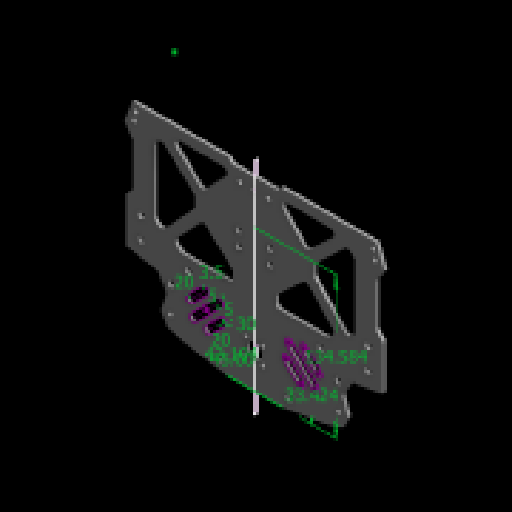
# Autodesk Inventor part: HeadMount
Saved by Autodesk Inventor 2025.2 (Build 292293000, 293)
## iProperties
Created: 2024-12-17
Part Number: HeadMount
Material: Generic
Document SubType Name: Sheet Metal
Designer: valer
Density: 1 g/cm^3
Sheet Metal Rule: Default
Appearance: Default
Author: valer
Autodesk Inventor part; units mm, degrees
ref_plane "YZ Plane" through (0, 0, 0) normal (1, 0, 0) x (0, 1, 0)
ref_plane "XZ Plane" through (0, 0, 0) normal (0, 1, 0) x (-1, 0, 0)
ref_plane "XY Plane" through (0, 0, 0) normal (0, 0, 1) x (1, 0, 0)
sketch "Sketch1" plane through (0, 0, 0) normal (0, 0, 1) x (1, 0, 0)
  circle A0 centre (-31.8464, -169.787) radius 2.7 construction
  circle A1 centre (-31.8464, -149.787) radius 2.7 construction
  arc A2 (-25.8464, -149.787) -> (-31.8464, -143.787) centre (-31.8464, -149.787) ccw construction
  line L0 (-31.8464, -143.787) -> (-53.675, -143.787) construction
  line L1 (-56.8232, -161.2642) -> (-53.675, -143.787) construction
  line L2 (-55.3879, -175.787) -> (-56.8232, -161.2642) construction
  line L3 (-55.3879, -175.787) -> (-31.8464, -175.787) construction
  arc A3 (-31.8464, -175.787) -> (-25.8464, -169.787) centre (-31.8464, -169.787) ccw construction
  line L4 (-25.8464, -169.787) -> (-25.8464, -149.787) construction
  circle A4 centre (183.4534, -169.787) radius 2.7 construction
  circle A5 centre (183.4534, -149.787) radius 2.7 construction
  arc A6 (183.4534, -143.787) -> (177.4534, -149.787) centre (183.4534, -149.787) ccw construction
  line L5 (177.4534, -169.787) -> (177.4534, -149.787) construction
  arc A7 (177.4534, -169.787) -> (183.4534, -175.787) centre (183.4534, -169.787) ccw construction
  line L6 (206.995, -175.787) -> (183.4534, -175.787) construction
  line L7 (206.995, -175.787) -> (208.4302, -161.2642) construction
  line L8 (208.4302, -161.2642) -> (205.282, -143.787) construction
  line L9 (183.4534, -143.787) -> (205.282, -143.787) construction
  line L10 (75.8035, -414.1995) -> (75.8035, 156.7514) construction
  line L11 (-46.34, -181.787) -> (-13.5242, -244.787)
  line L12 (-68.027, -161.7986) -> (-24.4397, -245.4777) construction
  line L13 (22.7981, -247.6758) -> (7.7102, -247.6758) construction
  circle A8 centre (22.7981, -241.6758) radius 2.7 construction
  circle A9 centre (22.7981, -223.6758) radius 2.7 construction
  circle A10 centre (22.7981, -223.6758) radius 3
  circle A11 centre (22.7981, -241.6758) radius 3
  circle A12 centre (-31.8464, -169.787) radius 3
  circle A13 centre (-31.8464, -149.787) radius 3
  line L14 (50.5095, -95.6646) -> (64.5095, -80.8626) construction
  line L15 (58.6334, -80.1159) -> (70.8035, -80.1159) construction
  circle A14 centre (37.042, -105.0395) radius 2.7 construction
  circle A15 centre (37.042, -117.0395) radius 2.7 construction
  circle A16 centre (114.5651, -105.0395) radius 2.7 construction
  circle A17 centre (114.5651, -117.0395) radius 2.7 construction
  circle A18 centre (128.8089, -223.6758) radius 2.7 construction
  circle A19 centre (128.8089, -241.6758) radius 2.7 construction
  line L16 (49.1565, -240.3427) -> (18.4758, -250.5451)
  line L17 (18.4758, -250.5451) -> (-13.5242, -244.787)
  line L18 (-39.6272, -91.7884) -> (-39.6272, -131.787)
  line L19 (-39.6272, -131.787) -> (-46.34, -139.787)
  line L20 (-46.34, -139.787) -> (-46.34, -181.787)
  line L21 (197.9471, -181.787) -> (165.1312, -244.787)
  circle A20 centre (128.8089, -223.6758) radius 3
  circle A21 centre (128.8089, -241.6758) radius 3
  circle A22 centre (183.4534, -169.787) radius 3
  circle A23 centre (183.4534, -149.787) radius 3
  line L22 (102.4505, -240.3427) -> (133.1312, -250.5451)
  line L23 (133.1312, -250.5451) -> (165.1312, -244.787)
  line L24 (191.2343, -91.7884) -> (191.2343, -131.787)
  line L25 (191.2343, -131.787) -> (197.9471, -139.787)
  line L26 (197.9471, -139.787) -> (197.9471, -181.787)
  circle A24 centre (-36.9593, -67.1208) radius 1.75 construction
  circle A25 centre (-38.635, -75.4158) radius 1.75 construction
  line L27 (-49.4079, -79.3835) -> (-42.2489, -59.9463) construction
  line L28 (-38.8427, -81.4928) -> (-49.4079, -79.3835) construction
  line L29 (-34.1095, -78.2645) -> (-38.8427, -81.4928) construction
  line L30 (-31.6784, -66.23) -> (-34.1095, -78.2645) construction
  line L31 (-34.7908, -61.4353) -> (-31.6784, -66.23) construction
  line L32 (-42.2489, -59.9463) -> (-34.7908, -61.4353) construction
  circle A26 centre (188.5664, -67.1208) radius 1.75 construction
  circle A27 centre (190.2421, -75.4158) radius 1.75 construction
  line L33 (193.8559, -59.9463) -> (201.0149, -79.3835) construction
  line L34 (186.3979, -61.4353) -> (193.8559, -59.9463) construction
  line L35 (183.2854, -66.23) -> (186.3979, -61.4353) construction
  line L36 (185.7165, -78.2645) -> (183.2854, -66.23) construction
  line L37 (190.4497, -81.4928) -> (185.7165, -78.2645) construction
  line L38 (201.0149, -79.3835) -> (190.4497, -81.4928) construction
  line L39 (-39.6272, -91.7884) -> (-47.4225, -79.7798)
  line L40 (-47.4225, -79.7798) -> (-40.2635, -60.3427)
  line L41 (-40.2635, -60.3427) -> (75.8035, -60.3427)
  line L42 (191.2343, -91.7884) -> (199.0296, -79.7798)
  line L43 (199.0296, -79.7798) -> (191.8706, -60.3427)
  line L44 (191.8706, -60.3427) -> (75.8035, -60.3427)
  line L45 (49.1565, -240.3427) -> (102.4505, -240.3427)
  circle A28 centre (-38.635, -75.4158) radius 2
  circle A29 centre (-36.9593, -67.1208) radius 2
  circle A30 centre (188.5664, -67.1208) radius 2
  circle A31 centre (190.2421, -75.4158) radius 2
  line L46 (-46.34, -181.787) -> (-15.2365, -187.3838)
  line L47 (-15.2365, -187.3838) -> (8.958, -233.8324)
  line L48 (8.958, -233.8324) -> (8.958, -248.8324)
  line L49 (197.9471, -181.787) -> (166.8435, -187.3838)
  line L50 (166.8435, -187.3838) -> (142.6491, -233.8324)
  line L51 (142.6491, -233.8324) -> (142.6491, -248.8324)
  line L52 (8.958, -233.8324) -> (49.1565, -240.3427)
  line L53 (102.4505, -240.3427) -> (142.6491, -233.8324)
  line L54 (142.6491, -233.8324) -> (158.8354, -228.7333)
  line L55 (158.8354, -228.7333) -> (164.3791, -218.0906)
  line L56 (164.3791, -218.0906) -> (159.28, -201.9042)
  line L57 (161.6073, -223.412) -> (150.9645, -217.8683) construction
  line L58 (8.958, -233.8324) -> (-7.2284, -228.7333)
  line L59 (-7.2284, -228.7333) -> (-12.7721, -218.0906)
  line L60 (-12.7721, -218.0906) -> (-7.673, -201.9042)
  point P0 (0, 0)
  point P1 (29.3253, -99.0395)
  point P2 (-39.6272, -132.4563)
  point P3 (-39.6272, -132.4563)
  dimension "d6" = 6
  dimension "d7" = 6
  dimension "d8" = 6
  dimension "d9" = 6
  dimension "d32" = 10
  dimension "d51" = 140
  dimension "d58" = 8
  dimension "d69" = 63
  dimension "d73" = 42
  dimension "d82" = 32
  dimension "d209" = 2
  dimension "d210" = 4
  dimension "d211" = 4
  dimension "d212" = 4
  dimension "d213" = 4
  dimension "d238" = 6
  dimension "d239" = 71.606
  dimension "d240" = 151.406
  dimension "d241" = 180
  dimension "d262" = 25
  dimension "d263" = 15
  dimension "d264" = 45
  dimension "d265" = 12
  dimension "d266" = 12
  measures "d6" diameter of A10
  measures "d7" diameter of A11
  measures "d8" diameter of A12
  measures "d9" diameter of A13
  measures "d32" distance between parallel lines of L11 L12
  measures "d51" angle of L20 L19
  measures "d58" vertical distance of L18.end L19.end
  measures "d69" vertical distance of L11.start L11.end
  measures "d73" distance of L19.end L11.start
  measures "d82" horizontal distance of L16.end L11.end
  measures "d209" distance between parallel lines of L27 L40
  measures "d210" diameter of A28
  measures "d211" diameter of A29
  measures "d212" diameter of A30
  measures "d213" diameter of A31
  measures "d238" distance from line of L3 L11.start
  measures "d239" angle of L16 L10
  measures "d240" angle of L16 L17
  measures "d241" distance between parallel lines of L45 L41
  measures "d262" distance between parallel lines of L11 L47
  measures "d263" distance of L47.end L48.end
  measures "d264" angle of L50 L54
  measures "d265" distance of L57.start L57.end
  measures "d266" distance of L54.end L55.end
extrude "Plate1" add sketch "Sketch1" along normal blind 3 contours L20 L19 L18 L39 L40 L41 L44 L43 L42 L24 L25 L26 L49 L50 L53 L45 L52 L47 L46 | L47 L58 L59 L60 | L50 L56 L55 L54 | A10 | A20
sketch "Sketch10" plane through (0, 0, 3) normal (0, 0, 1) x (1, 0, 0)
  arc A0 (76.8035, -214.1927) -> (74.8035, -214.1927) centre (75.8035, -207.2645) ccw construction
  circle A1 centre (75.8035, -207.2645) radius 7
  line L0 (45.7546, -229.3135) -> (45.0245, -232.0574) construction
  arc A2 (45.7546, -229.3135) -> (45.0245, -232.0574) centre (42.9736, -230.0426) ccw construction
  arc A3 (106.1334, -231.4623) -> (106.1334, -228.6229) centre (108.6334, -230.0426) ccw construction
  circle A4 centre (42.9736, -230.0426) radius 3.1
  circle A5 centre (108.6334, -230.0426) radius 3.1
  arc A6 (-1.2619, -190.9216) -> (-1.2619, -193.761) centre (-3.7619, -192.3413) ccw construction
  arc A7 (15.5855, -171.9674) -> (15.5855, -174.8068) centre (13.0855, -173.3871) ccw construction
  arc A8 (136.0216, -174.8068) -> (136.0216, -171.9674) centre (138.5216, -173.3871) ccw construction
  arc A9 (152.8689, -193.761) -> (152.8689, -190.9216) centre (155.3689, -192.3413) ccw construction
  arc A10 (-1.2619, -190.9216) -> (-1.2619, -193.761) centre (-3.7619, -192.3413) ccw projected
  circle A11 centre (-3.7619, -192.3413) radius 3.1
  arc A12 (15.5855, -171.9674) -> (15.5855, -174.8068) centre (13.0855, -173.3871) ccw projected
  circle A13 centre (13.0855, -173.3871) radius 3.1
  arc A14 (136.0216, -174.8068) -> (136.0216, -171.9674) centre (138.5216, -173.3871) ccw projected
  circle A15 centre (138.5216, -173.3871) radius 3.1
  circle A16 centre (155.3689, -192.3413) radius 3.1
  arc A17 (69.2244, -198.4257) -> (66.5765, -198.1614) centre (67.8035, -199.2645) ccw construction
  arc A18 (85.7112, -198.6639) -> (85.5795, -200.1843) centre (83.8035, -199.2645) ccw construction
  arc A19 (65.8958, -215.8651) -> (66.0276, -214.3447) centre (67.8035, -215.2645) ccw construction
  arc A20 (84.4041, -217.1722) -> (82.8838, -217.0405) centre (83.8035, -215.2645) ccw construction
  circle A21 centre (67.8035, -199.2645) radius 2.1
  circle A22 centre (83.8035, -199.2645) radius 2.1
  circle A23 centre (83.8035, -215.2645) radius 2.1
  circle A24 centre (67.8035, -215.2645) radius 2.1
  point P0 (0, 0)
  dimension "d150" = 6.2
  dimension "d153" = 4.2
  constraints: 11 coincident, 10 centre point, 8 equal radius, 3 other
  measures "d150" diameter of A4
  measures "d153" diameter of A21
extrude "Extrusion5" cut sketch "Sketch10" against normal through all
sketch "Sketch11" plane through (0, 0, 3) normal (0, 0, 1) x (1, 0, 0)
  line L0 (42.8154, -184.2567) -> (17.679, -209.3932) construction
  line L1 (40.3405, -181.7819) -> (15.2041, -206.9183)
  line L2 (20.1538, -211.868) -> (45.2903, -186.7316)
  arc A0 (45.2903, -186.7316) -> (40.3405, -181.7819) centre (42.8154, -184.2567) ccw
  arc A1 (15.2041, -206.9183) -> (20.1538, -211.868) centre (17.679, -209.3932) ccw
  line L3 (45.8035, -198.2392) -> (31.6614, -212.3813) construction
  line L4 (43.3286, -195.7643) -> (29.1865, -209.9064)
  line L5 (34.1363, -214.8562) -> (48.2784, -200.714)
  arc A2 (48.2784, -200.714) -> (43.3286, -195.7643) centre (45.8035, -198.2392) ccw
  arc A3 (29.1865, -209.9064) -> (34.1363, -214.8562) centre (31.6614, -212.3813) ccw
  line L6 (28.833, -181.2686) -> (14.6908, -195.4107) construction
  line L7 (31.3078, -183.7435) -> (17.1657, -197.8856)
  line L8 (12.2159, -192.9359) -> (26.3581, -178.7937)
  arc A4 (31.3078, -183.7435) -> (26.3581, -178.7937) centre (28.833, -181.2686) ccw
  arc A5 (12.2159, -192.9359) -> (17.1657, -197.8856) centre (14.6908, -195.4107) ccw
  line L9 (75.8035, -105.7591) -> (75.8035, -240.3427) construction
  line L10 (21.7619, -188.3397) -> (38.7325, -205.3102) construction
  line L11 (111.2665, -181.7819) -> (136.403, -206.9183)
  line L12 (131.4532, -211.868) -> (106.3168, -186.7316)
  arc A6 (111.2665, -181.7819) -> (106.3168, -186.7316) centre (108.7917, -184.2567) ccw
  arc A7 (131.4532, -211.868) -> (136.403, -206.9183) centre (133.9281, -209.3932) ccw
  line L13 (108.2784, -195.7643) -> (122.4205, -209.9064)
  line L14 (117.4708, -214.8562) -> (103.3286, -200.714)
  arc A8 (108.2784, -195.7643) -> (103.3286, -200.714) centre (105.8035, -198.2392) ccw
  arc A9 (117.4708, -214.8562) -> (122.4205, -209.9064) centre (119.9457, -212.3813) ccw
  line L15 (120.2992, -183.7435) -> (134.4413, -197.8856)
  line L16 (139.3911, -192.9359) -> (125.249, -178.7937)
  arc A10 (125.249, -178.7937) -> (120.2992, -183.7435) centre (122.7741, -181.2686) ccw
  arc A11 (134.4413, -197.8856) -> (139.3911, -192.9359) centre (136.9162, -195.4107) ccw
  line L17 (102.4505, -240.3427) -> (49.1565, -240.3427) projected
  point P0 (0, 0)
  point P1 (30.2472, -196.8249)
  dimension "d154" = 3.5
  dimension "d155" = 5
  dimension "d156" = 5
  dimension "d163" = 30
  dimension "d165" = 20
  dimension "d214" = 45
  dimension "d215" = 42.1035
  dimension "d217" = 33.4244
  dimension "d218" = 134.5835
  dimension "d242" = 20
  constraints: 40 end point, 24 point on circle, 18 symmetric about line, 12 centre point, 12 tangent, 5 midpoint, 5 parallel, 2 equal radius, 2 perpendicular, 6 other
  measures "d154" radius of A4
  measures "d155" distance between parallel lines of L1 L7
  measures "d156" distance between parallel lines of L4 L2
  measures "d163" distance from line of L9 L3.start
  measures "d165" distance of L6.start L6.end
  measures "d214" angle of L17 L3
  measures "d215" distance from line of L17 L3.start
  measures "d217" distance from line of L11.end L17
  measures "d218" distance from line of L9.start L17
  measures "d242" distance of L3.start L3.end
extrude "Extrusion6" cut sketch "Sketch11" against normal through all
sketch "Sketch13" plane through (0, 0, 3) normal (0, 0, 1) x (1, 0, 0)
  circle A0 centre (62.3035, -56.7429) radius 2 construction
  circle A1 centre (89.3035, -56.7429) radius 2 construction
  line L0 (98.1778, -70.2429) -> (53.4293, -70.2429) construction
  line L1 (75.8035, -70.2429) -> (75.8035, -80.2429) construction
  line L2 (53.4293, -70.2429) -> (53.4293, -80.2429) construction
  line L3 (53.4293, -75.2429) -> (75.8035, -75.2429) construction
  line L4 (62.3035, -56.7429) -> (62.3035, -75.2429) construction
  circle A2 centre (62.3035, -75.2429) radius 2
  circle A3 centre (75.8035, -75.2429) radius 2
  circle A4 centre (89.3035, -75.2429) radius 2
  point P0 (0, 0)
  dimension "d174" = 4
  dimension "d175" = 4
  constraints: 10 end point, 3 centre point, 3 midpoint, 2 coincident, 1 perpendicular, 1 point on line, 1 symmetric about line, 1 vertical, 1 other
  measures "d174" diameter of A2
  measures "d175" diameter of A3
extrude "Cut1" cut sketch "Sketch13" against normal blind 3
fillet "Fillet1" radius 2 20 edges at (-39.6272, -91.7884, 1.5) (-39.6272, -131.787, 1.5) (-46.34, -139.787, 1.5) (-46.34, -181.787, 1.5) (49.1565, -240.3427, 1.5) (102.4505, -240.3427, 1.5) (197.9471, -181.787, 1.5) (197.9471, -139.787, 1.5) (191.2343, -131.787, 1.5) (191.2343, -91.7884, 1.5) (-15.2365, -187.3838, 1.5) (8.958, -233.8324, 1.5) (166.8435, -187.3838, 1.5) (142.6491, -233.8324, 1.5) (-7.673, -201.9042, 1.5) (-12.7721, -218.0906, 1.5) (-7.2284, -228.7333, 1.5) (159.28, -201.9042, 1.5) (164.3791, -218.0906, 1.5) (158.8354, -228.7333, 1.5)
sketch "Sketch17" plane through (0, 0, 3) normal (0, 0, 1) x (1, 0, 0)
  line L0 (44.5586, -95.6074) -> (52.8519, -81.2429)
  arc A0 (54.584, -80.2429) -> (52.8519, -81.2429) centre (54.584, -82.2429) ccw
  line L1 (54.584, -80.2429) -> (97.023, -80.2429)
  arc A1 (98.7551, -81.2429) -> (97.023, -80.2429) centre (97.023, -82.2429) ccw
  line L2 (98.7551, -81.2429) -> (107.0485, -95.6074)
  arc A2 (107.269, -97.0403) -> (107.0485, -95.6074) centre (105.3164, -96.6074) ccw
  line L3 (106.3291, -101.28) -> (107.269, -97.0403)
  arc A3 (105.5236, -102.4855) -> (106.3291, -101.28) centre (104.3765, -100.8471) ccw
  line L4 (105.5236, -102.4855) -> (98.5318, -107.3812)
  arc A4 (97.3847, -107.7429) -> (98.5318, -107.3812) centre (97.3847, -105.7429) ccw
  line L5 (97.3847, -107.7429) -> (54.2224, -107.7429)
  arc A5 (53.0752, -107.3812) -> (54.2224, -107.7429) centre (54.2224, -105.7429) ccw
  line L6 (53.0752, -107.3812) -> (46.0834, -102.4855)
  arc A6 (45.278, -101.28) -> (46.0834, -102.4855) centre (47.2306, -100.8471) ccw
  line L7 (44.338, -97.0403) -> (45.278, -101.28)
  arc A7 (44.5586, -95.6074) -> (44.338, -97.0403) centre (46.2906, -96.6074) ccw
  point P0 (0, 0)
sheet face with bend "Face6" sketch "Sketch17" thickness 3 toward (0, 0, -1) bend radius 3 relief straight relief width 3 relief depth 1.5
bend "Bend5"
sketch "Sketch18" plane through (0, 0, 3) normal (0, 0, 1) x (1, 0, 0)
  line L0 (4.6693, -117.8173) -> (9.4448, -115.0601)
  arc A0 (10.4448, -114.7922) -> (9.4448, -115.0601) centre (10.4448, -116.7922) ccw
  line L1 (10.4448, -114.7922) -> (17.373, -114.7922)
  arc A1 (18.373, -115.0601) -> (17.373, -114.7922) centre (17.373, -116.7922) ccw
  arc A2 (4.6693, -117.8173) -> (3.7838, -118.8824) centre (5.6693, -119.5493) ccw
  line L2 (3.7838, -118.8824) -> (2.248, -123.2238)
  arc A3 (2.248, -123.2238) -> (2.2668, -124.6088) centre (4.1335, -123.8908) ccw
  line L3 (16.2921, -161.0744) -> (2.2668, -124.6088)
  line L4 (18.373, -115.0601) -> (45.611, -130.786)
  arc A4 (46.611, -132.5181) -> (45.611, -130.786) centre (44.611, -132.5181) ccw
  line L5 (46.611, -132.5181) -> (46.611, -148.4861)
  arc A5 (46.611, -148.4861) -> (47.2565, -149.9575) centre (48.611, -148.4861) ccw
  line L6 (47.2565, -149.9575) -> (59.7731, -161.4802)
  arc A6 (60.4142, -163.082) -> (59.7731, -161.4802) centre (58.4185, -162.9516) ccw
  line L7 (60.4142, -163.082) -> (59.8495, -171.7285)
  arc A7 (59.3252, -172.9527) -> (59.8495, -171.7285) centre (57.8538, -171.5981) ccw
  line L8 (59.3252, -172.9527) -> (57.0902, -175.3806)
  arc A8 (55.7014, -176.0243) -> (57.0902, -175.3806) centre (55.6187, -174.026) ccw
  line L9 (51.7048, -176.1895) -> (55.7014, -176.0243)
  arc A9 (50.2676, -175.6627) -> (51.7048, -176.1895) centre (51.6222, -174.1912) ccw
  line L10 (50.2676, -175.6627) -> (39.6798, -165.9157)
  arc A10 (39.6798, -165.9157) -> (38.3252, -165.3871) centre (38.3252, -167.3871) ccw
  line L11 (38.3252, -165.3871) -> (22.5715, -165.3871)
  arc A11 (21.4392, -165.0357) -> (22.5715, -165.3871) centre (22.5715, -163.3871) ccw
  line L12 (17.0265, -162.0051) -> (21.4392, -165.0357)
  arc A12 (16.2921, -161.0744) -> (17.0265, -162.0051) centre (18.1588, -160.3565) ccw
  arc A13 (91.834, -161.4802) -> (91.1928, -163.082) centre (93.1886, -162.9516) ccw
  line L13 (91.834, -161.4802) -> (104.3506, -149.9575)
  line L14 (91.7575, -171.7285) -> (91.1928, -163.082)
  arc A14 (91.7575, -171.7285) -> (92.2818, -172.9527) centre (93.7532, -171.5981) ccw
  line L15 (94.5169, -175.3806) -> (92.2818, -172.9527)
  arc A15 (94.5169, -175.3806) -> (95.9057, -176.0243) centre (95.9883, -174.026) ccw
  line L16 (95.9057, -176.0243) -> (99.9023, -176.1895)
  arc A16 (99.9023, -176.1895) -> (101.3395, -175.6627) centre (99.9849, -174.1912) ccw
  line L17 (111.9273, -165.9157) -> (101.3395, -175.6627)
  arc A17 (113.2818, -165.3871) -> (111.9273, -165.9157) centre (113.2818, -167.3871) ccw
  line L18 (129.0355, -165.3871) -> (113.2818, -165.3871)
  arc A18 (129.0355, -165.3871) -> (130.1678, -165.0357) centre (129.0355, -163.3871) ccw
  line L19 (130.1678, -165.0357) -> (134.5805, -162.0051)
  arc A19 (134.5805, -162.0051) -> (135.3149, -161.0744) centre (133.4482, -160.3565) ccw
  line L20 (149.3402, -124.6088) -> (135.3149, -161.0744)
  arc A20 (149.3402, -124.6088) -> (149.359, -123.2238) centre (147.4735, -123.8908) ccw
  line L21 (149.359, -123.2238) -> (147.8233, -118.8824)
  arc A21 (147.8233, -118.8824) -> (146.9378, -117.8173) centre (145.9378, -119.5493) ccw
  line L22 (142.1622, -115.0601) -> (146.9378, -117.8173)
  arc A22 (142.1622, -115.0601) -> (141.1622, -114.7922) centre (141.1622, -116.7922) ccw
  line L23 (134.234, -114.7922) -> (141.1622, -114.7922)
  arc A23 (134.234, -114.7922) -> (133.234, -115.0601) centre (134.234, -116.7922) ccw
  line L24 (105.996, -130.786) -> (133.234, -115.0601)
  arc A24 (105.996, -130.786) -> (104.996, -132.5181) centre (106.996, -132.5181) ccw
  line L25 (104.996, -148.4861) -> (104.996, -132.5181)
  arc A25 (104.3506, -149.9575) -> (104.996, -148.4861) centre (102.996, -148.4861) ccw
  point P0 (0, 0)
sheet face with bend "Face7" sketch "Sketch18" thickness 3 toward (0, 0, -1) bend radius 3 relief straight relief width 3 relief depth 1.5
bend "Bend6"
sketch "Sketch19" plane through (0, 0, 3) normal (0, 0, 1) x (1, 0, 0)
  line L0 (191.8706, -60.3427) -> (-40.2635, -60.3427) projected
  line L1 (50.9033, -60.3427) -> (54.8035, -64.2429)
  line L2 (54.8035, -64.2429) -> (96.8035, -64.2429)
  line L3 (96.8035, -64.2429) -> (100.7037, -60.3427)
  line L4 (75.8035, -64.2429) -> (75.8035, -60.3427)
  line L5 (-40.2635, -60.3427) -> (191.8706, -60.3427) projected
  line L6 (96.8035, -64.2429) -> (54.8035, -64.2429) projected
  point P0 (0, 0)
  constraints: 8 end point, 3 perpendicular, 2 midpoint, 2 point on line, 1 collinear, 1 parallel
extrude "Cut3" cut sketch "Sketch19" against normal blind 3
sketch "Sketch20" plane through (0, 0, 3) normal (0, 0, 1) x (1, 0, 0)
  line L0 (-5.9873, -70.3427) -> (54.8035, -70.3427)
  line L1 (54.8035, -70.3427) -> (26.5284, -100.664)
  line L2 (-5.9873, -70.3427) -> (26.5284, -100.664)
  line L3 (19.7084, -107.9776) -> (19.7084, -117.9776)
  line L4 (19.7084, -117.9776) -> (-12.3137, -152.3171)
  line L5 (54.8035, -64.2429) -> (50.9033, -60.3427) projected
  line L6 (-40.2635, -60.3427) -> (50.9033, -60.3427) projected
  line L7 (-39.6272, -131.059) -> (-39.6272, -92.3806) projected
  line L8 (-46.34, -180.1147) -> (-46.34, -140.5149) projected
  line L9 (-45.8721, -139.2293) -> (-40.0951, -132.3446) projected
  line L10 (-39.9497, -91.2916) -> (-47.4225, -79.7798) projected
  line L11 (-47.4225, -79.7798) -> (-40.2635, -60.3427) projected
  line L12 (-0.9715, -154.8168) -> (27.022, -124.7976)
  line L13 (55.8035, -161.6368) -> (6.3421, -161.6368)
  line L14 (6.3421, -161.6368) -> (-0.9715, -154.8168)
  line L15 (27.022, -124.7976) -> (55.8035, -151.6368)
  line L16 (55.8035, -151.6368) -> (55.8035, -161.6368)
  line L17 (54.8035, -64.2429) -> (96.8035, -64.2429) projected
  line L18 (75.8035, -64.2429) -> (75.8035, -240.3427) construction
  line L19 (49.3174, -240.3427) -> (102.2896, -240.3427) projected
  line L20 (157.5943, -70.3427) -> (96.8035, -70.3427)
  line L21 (96.8035, -70.3427) -> (125.0786, -100.664)
  line L22 (157.5943, -70.3427) -> (125.0786, -100.664)
  line L23 (152.5785, -154.8168) -> (124.5851, -124.7976)
  line L24 (95.8035, -161.6368) -> (145.265, -161.6368)
  line L25 (145.265, -161.6368) -> (152.5785, -154.8168)
  line L26 (124.5851, -124.7976) -> (95.8035, -151.6368)
  line L27 (95.8035, -151.6368) -> (95.8035, -161.6368)
  line L28 (42.3861, -118.6149) -> (75.8035, -149.7772)
  line L29 (75.8035, -149.7772) -> (109.221, -118.6149)
  line L30 (42.3861, -118.6149) -> (109.221, -118.6149) construction
  line L31 (42.3861, -105.653) -> (62.3513, -84.2429)
  line L32 (62.3513, -84.2429) -> (89.2557, -84.2429)
  line L33 (89.2557, -84.2429) -> (109.221, -105.653)
  line L34 (109.221, -105.653) -> (42.3861, -105.653) construction
  line L35 (42.3861, -105.653) -> (42.3861, -118.6149)
  line L36 (109.221, -105.653) -> (109.221, -118.6149)
  line L37 (-5.9873, -70.3427) -> (-12.8073, -77.6562) construction
  line L38 (-19.6272, -84.9698) -> (-19.6272, -145.4971)
  line L39 (-19.6272, -145.4971) -> (-12.3137, -152.3171)
  line L40 (-12.8073, -77.6562) -> (-19.6272, -84.9698)
  line L41 (-12.8073, -77.6562) -> (19.7084, -107.9776)
  line L42 (131.8986, -107.9776) -> (131.8986, -117.9776)
  line L43 (131.8986, -117.9776) -> (163.9207, -152.3171)
  line L44 (171.2343, -84.9698) -> (171.2343, -145.4971)
  line L45 (171.2343, -145.4971) -> (163.9207, -152.3171)
  line L46 (164.4143, -77.6562) -> (171.2343, -84.9698)
  line L47 (164.4143, -77.6562) -> (131.8986, -107.9776)
  line L48 (26.5284, -100.664) -> (19.7084, -107.9776) construction
  line L49 (27.022, -124.7976) -> (19.7084, -117.9776) construction
  line L50 (54.8035, -70.3427) -> (54.8035, -64.2429) construction
  line L51 (96.8035, -64.2429) -> (54.8035, -64.2429) projected
  point P0 (0, 0)
  point P1 (75.8035, -105.653)
  dimension "d221" = 10
  dimension "d243" = 22.6776
  dimension "d244" = 10
  dimension "d245" = 15
  dimension "d246" = 20
  dimension "d247" = 47
  dimension "d248" = 15
  dimension "d249" = 10
  dimension "d250" = 20
  dimension "d251" = 10
  dimension "d252" = 10
  dimension "d253" = 20
  dimension "d254" = 10
  dimension "d255" = 10
  dimension "d256" = 133
  dimension "d257" = 133
  dimension "d258" = 10
  constraints: 84 end point, 15 symmetric about line, 11 parallel, 10 perpendicular, 3 midpoint, 2 point on line, 2 vertical, 1 collinear, 1 horizontal
  measures "d221" distance between parallel lines of L6 L0
  measures "d243" distance between parallel lines of L35 L3
  measures "d244" distance between parallel lines of L41 L2
  measures "d245" distance between parallel lines of L31 L1
  measures "d246" distance between parallel lines of L17 L32
  measures "d247" angle of L1 L0
  measures "d248" distance between parallel lines of L28 L15
  measures "d249" distance between parallel lines of L12 L4
  measures "d250" distance between parallel lines of L7 L38
  measures "d251" distance of L37.end L38.start
  measures "d252" distance of L13.end L12.start
  measures "d253" distance between parallel lines of L18 L16
  measures "d254" distance of L15.end L13.start
  measures "d255" distance of L3.start L3.end
  measures "d256" angle of L32 L31
  measures "d257" angle of L33 L32
  measures "d258" distance of L38.end L4.end
extrude "Cut4" cut sketch "Sketch20" against normal blind 3 contours L0 L1 L2 | L3 L4 L39 L38 L40 L41 | L12 L15 L16 L13 L14 | L22 L21 L20 | L25 L24 L27 L26 L23 | L47 L46 L44 L45 L43 L42
fillet "Fillet5" radius 4 28 edges at (54.8035, -70.3427, 1.5) (-5.9873, -70.3427, 1.5) (26.5284, -100.664, 1.5) (-12.8073, -77.6562, 1.5) (-19.6272, -84.9698, 1.5) (-19.6272, -145.4971, 1.5) (-12.3137, -152.3171, 1.5) (19.7084, -117.9776, 1.5) (19.7084, -107.9776, 1.5) (-0.9715, -154.8168, 1.5) (27.022, -124.7976, 1.5) (55.8035, -161.6368, 1.5) (55.8035, -151.6368, 1.5) (6.3421, -161.6368, 1.5) (96.8035, -70.3427, 1.5) (157.5943, -70.3427, 1.5) (125.0786, -100.664, 1.5) (171.2343, -84.9698, 1.5) (164.4143, -77.6562, 1.5) (131.8986, -107.9776, 1.5) (131.8986, -117.9776, 1.5) (163.9207, -152.3171, 1.5) (171.2343, -145.4971, 1.5) (124.5851, -124.7976, 1.5) (95.8035, -151.6368, 1.5) (95.8035, -161.6368, 1.5) (145.265, -161.6368, 1.5) (152.5785, -154.8168, 1.5)
ref_plane "MidPlane" through (75.8035, -116.4019, 3) normal (-1, 0, 0) x (0, 0, 1)
sketch "Sketch22" plane through (0, 0, 3) normal (0, 0, 1) x (1, 0, 0)
  circle A0 centre (-4.1461, -217.3337) radius 2
  line L0 (96.8035, -64.2429) -> (54.8035, -64.2429) projected
  line L1 (102.2896, -240.3427) -> (49.3174, -240.3427) projected
  line L2 (54.8035, -64.2429) -> (96.8035, -64.2429) projected
  line L3 (75.8035, -64.2429) -> (75.8035, -240.3427)
  circle A1 centre (155.7531, -217.3337) radius 2
  line L4 (-7.6111, -227.9986) -> (-12.3894, -218.8253) projected
  line L5 (-12.5232, -217.3005) -> (-7.9219, -202.6944) projected
  point P0 (0, 0)
  dimension "d267" = 4
  dimension "d268" = 8
  dimension "d269" = 8
  constraints: 2 centre point, 2 end point, 2 midpoint, 1 symmetric about line, 1 other
  measures "d267" diameter of A0
  measures "d268" distance from line of L4 A0.centre
  measures "d269" distance from line of L5 A0.centre
extrude "Cut6" cut sketch "Sketch22" against normal blind 3
sketch "Sketch24" plane through (0, 0, 3) normal (0, 0, 1) x (1, 0, 0)
  circle A0 centre (60.8035, -115.7754) radius 3 projected
  circle A1 centre (60.8035, -129.1754) radius 3 projected
  circle A2 centre (90.8035, -115.7754) radius 3 projected
  circle A3 centre (90.8035, -129.1754) radius 3 projected
  point P0 (0, 0)
extrude "Cut8" cut sketch "Sketch24" against normal blind 3
equation "\"d7\" = d6"
equation "\"d8\" = d6"
equation "\"d9\" = d6"
equation "\"d1\" = Thickness"
equation "\"BendRadius\" = Thickness"
equation "\"BendReliefWidth\" = Thickness"
equation "\"BendReliefDepth\" = 0.5 * Thickness"
equation "\"CornerReliefSize\" = 4 * Thickness"
equation "\"MinimumRemnant\" = 2 * Thickness"
equation "\"TransitionRadius\" = BendRadius"
equation "\"JacobiRadiusSize\" = BendRadius"
equation "\"GapSize\" = Thickness"
equation "\"Thickness\" = 3"
body "Solid1"
